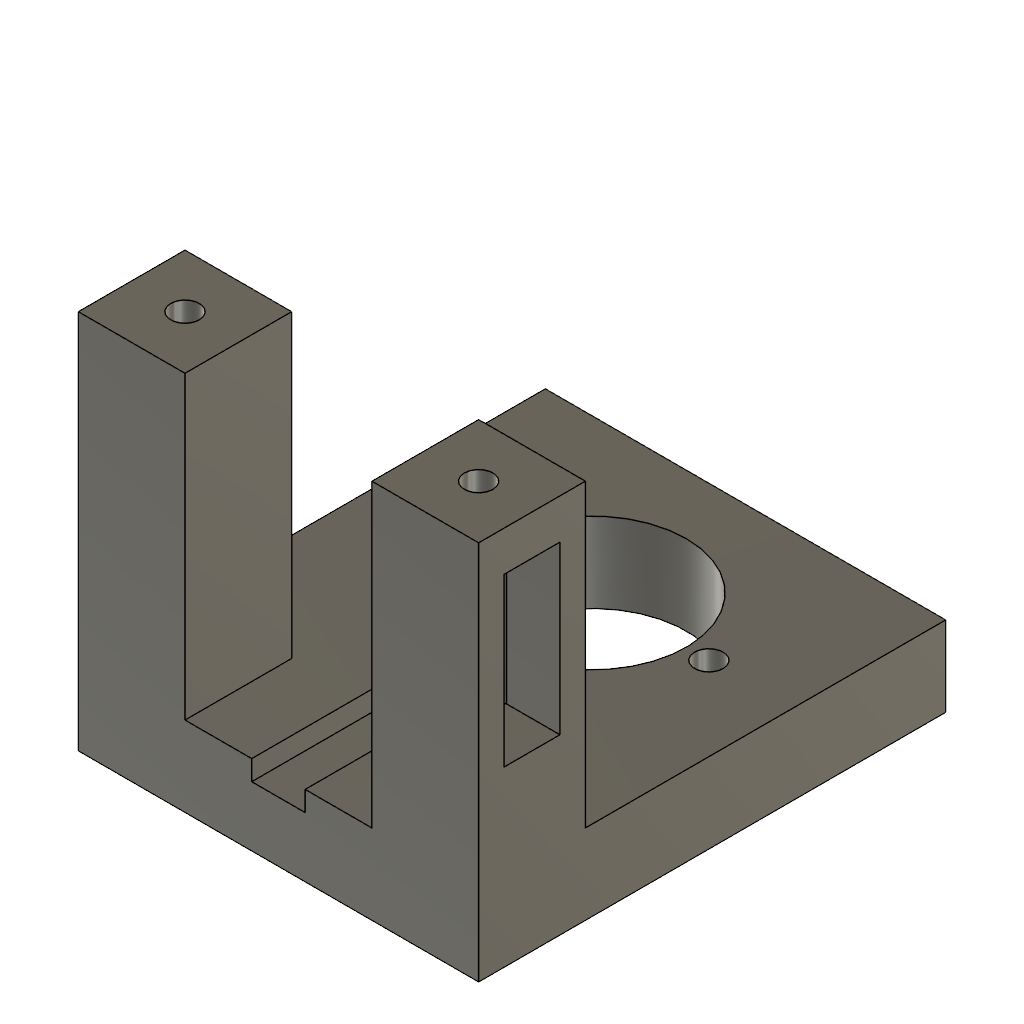
05 - PRIMARY SUPPORT MECHANISM ( LEFT SIDE ) (Autodesk Fusion 360 design; units mm, degrees)
Autodesk Fusion 360 part; units mm, degrees
sketch "01 - PRIMARY SUPPORT MECHANISM ( LEFT SIDE ) SKETCH" plane through (0, 0, 0) normal (0, 0, 1) x (1, 0, 0)
  line L0 (0, -35) -> (0, -5.422) construction
  line L1 (13.875, 9.9067) -> (17.5, 7.8138)
  circle A0 centre (17.5, 11.9996) radius 2.14
  line L2 (-13.875, 14.0925) -> (-17.5, 16.1854)
  circle A1 centre (-17.5, 11.9996) radius 2.14
  line L3 (-21.125, 14.0925) -> (-21.125, 9.9067)
  line L4 (4, -5.422) -> (4, -35)
  line L5 (30, 35) -> (30, -35)
  line L6 (-7.6, -5.422) -> (-7.6, 0.1231)
  line L7 (-4, -5.422) -> (-4, -35)
  line L8 (17.5, 7.8138) -> (21.125, 9.9067)
  line L9 (-21.125, 9.9067) -> (-17.5, 7.8138)
  line L10 (7.6, -5.422) -> (7.6, 0.1231)
  line L11 (21.125, 14.0925) -> (17.5, 16.1854)
  line L12 (-30, 35) -> (30, 35)
  line L13 (21.125, 9.9067) -> (21.125, 14.0925)
  line L14 (13.875, 14.0925) -> (13.875, 9.9067)
  line L15 (-17.5, 7.8138) -> (-13.875, 9.9067)
  line L16 (-30, -19) -> (30, -19) construction
  line L17 (30, -35) -> (-30, -35)
  line L18 (17.5, 16.1854) -> (13.875, 14.0925)
  line L19 (-17.5, 11.9996) -> (-17.5, 14.1396) construction
  line L20 (17.5, 11.9996) -> (17.5, 14.1396) construction
  line L21 (-17.5, 11.9996) -> (17.5, 11.9996) construction
  arc A2 (7.6, 0.1231) -> (-7.6, 0.1231) centre (0, 11.9996) ccw
  line L22 (-17.5, 16.1854) -> (-21.125, 14.0925)
  line L23 (-30, -35) -> (-30, 35)
  line L24 (-7.6, -5.422) -> (7.6, -5.422)
  line L25 (-13.875, 9.9067) -> (-13.875, 14.0925)
  point P0 (17.5, 11.9996)
  point P1 (-17.5, 11.9996)
  dimension "d1" = 60
  dimension "d2" = 70
  dimension "d5" = 16
  dimension "d6" = 29.578
  dimension "d7" = 15.2
  dimension "d8" = 5.5451
  dimension "d9" = 14.1
  dimension "d10" = 17.4216
  dimension "d11" = 8
  dimension "d12" = 4
  dimension "d13" = 35
  dimension "d14" = 4.28
  dimension "d15" = 3.625
  dimension "d16" = 4.28
  dimension "d17" = 3.625
  dimension "d19" = 35
  dimension "d20" = 30
  constraint horizontal L12
  constraint vertical L5
  constraint horizontal L17
  constraint vertical L23
  constraint coincident L16.start L23
  constraint coincident L16.end L5
  constraint perpendicular L5 L16
  constraint midpoint L0.start L17
  constraint perpendicular L0 L16
  constraint equal L6 L10
  constraint parallel L6 L10
  constraint perpendicular L10 L24
  constraint coincident L0.end L24
  constraint midpoint L0.end L24
  constraint horizontal L24
  constraint coincident L4.start L24
  constraint coincident L4.end L17
  constraint perpendicular L4 L17
  constraint coincident L7.start L24
  constraint coincident L7.end L17
  constraint perpendicular L7 L17
  constraint horizontal L21
  constraint midpoint A2.centre L21
  constraint coincident P0 A0.centre
  constraint coincident L20.end A0
  constraint perpendicular L20 L21
  constraint coincident L11.end L20
  constraint coincident P1 A1.centre
  constraint coincident L19.end A1
  constraint perpendicular L19 L21
  constraint coincident L2.end L19
  measures "d1" distance of L5.start L12.start
  measures "d2" distance of L12.start L17.end
  measures "d5" distance of L16 L17
  measures "d6" distance of L0.start L0.end
  measures "d7" distance of L10.start L6.start
  measures "d8" distance of L10.end L10.start
  measures "d9" radius of A2
  measures "d10" distance of A2.centre L24
  measures "d11" distance of L4 L7
  measures "d12" distance of L0 L7
  measures "d13" horizontal distance of P1 P0
  measures "d14" diameter of A0
  measures "d15" distance of P0 L13
  measures "d16" diameter of A1
  measures "d17" distance of P1 L15
  measures "d19" distance of origin L12
  measures "d20" distance of origin L23
  measures "d38" distance of L4.start
extrude "Extrude1" add sketch "01 - PRIMARY SUPPORT MECHANISM ( LEFT SIDE ) SKETCH" along normal blind 12 contours L1 L8 L11 L13 L18 A2 | L1 L2 L3 L4 L5 L6 L7 L8 L9 L10 L11 L12 L13 L15 L17 L18 A2 L22 L23 L24 | L2 L3 L9 L15 A2 L22 | A0 | A1
extrude "Extrude2" add sketch "01 - PRIMARY SUPPORT MECHANISM ( LEFT SIDE ) SKETCH" along normal blind 9 contours L4 L7 L17 L24
sketch "02 - PRIMARY SUPPORT MECHANISM ( LEFT SIDE ) SKETCH" plane through (0, 0, 12) normal (0, 0, 1) x (-1, 0, 0)
  line L0 (-4, 5.422) -> (-4, 35)
  line L1 (-4, 35) -> (-30, 35)
  line L2 (-30, 35) -> (-30, -35)
  line L3 (-30, -35) -> (30, -35)
  line L4 (30, -35) -> (30, 35)
  line L5 (30, 35) -> (4, 35)
  line L6 (4, 35) -> (4, 5.422)
  line L7 (4, 5.422) -> (7.6, 5.422)
  line L8 (7.6, 5.422) -> (7.6, -0.1231)
  arc A0 (-7.6, -0.1231) -> (7.6, -0.1231) centre (0, -11.9996) ccw
  line L9 (-7.6, -0.1231) -> (-7.6, 5.422)
  line L10 (-7.6, 5.422) -> (-4, 5.422)
  line L11 (30, 35) -> (4, 35)
  line L12 (-4, 35) -> (-30, 35)
  line L13 (30, 35) -> (14, 35)
  line L14 (-14, 35) -> (-14, 19)
  line L15 (14, 35) -> (14, 19)
  line L16 (-30, 19) -> (-30, 35)
  line L17 (-30, 35) -> (-14, 35)
  line L18 (30, 19) -> (30, 35)
  line L19 (14, 19) -> (30, 19)
  line L20 (-14, 19) -> (-30, 19)
  dimension "d25" = 16
  dimension "d26" = 16
  dimension "d27" = 16
  dimension "d28" = 16
  constraint horizontal L13
  constraint vertical L15
  constraint horizontal L19
  constraint vertical L18
  constraint coincident L4.end L5.start
  constraint horizontal L17
  constraint vertical L14
  constraint horizontal L20
  constraint vertical L16
  constraint coincident L1.end L2.start
  constraint coincident L5.end L6.start
  constraint coincident L0.end L1.start
  measures "d25" distance of L13.end L4.end
  measures "d26" distance of L18.start L4.end
  measures "d27" distance of L14.start L1.end
  measures "d28" distance of L1.end L16.start
extrude "Extrude3" add sketch "02 - PRIMARY SUPPORT MECHANISM ( LEFT SIDE ) SKETCH" along normal blind 45 contours L1 L2 L12 L14 L16 L17 L20 | L4 L5 L11 L13 L15 L18 L19
sketch "03 - PRIMARY SUPPORT MECHANISM ( LEFT SIDE ) SKETCH" plane through (0, 0, 57) normal (0, 0, 1) x (-1, 0, 0)
  line L0 (-14, 19) -> (-14, 35)
  line L1 (-14, 35) -> (-30, 35)
  line L2 (-30, 35) -> (-30, 19)
  line L3 (-30, 19) -> (-14, 19)
  line L4 (-14, 35) -> (-30, 35)
  line L5 (-18.375, 29.0929) -> (-22, 31.1858)
  line L6 (-14, 19) -> (-14, 35)
  line L7 (-22, 22.8142) -> (-18.375, 24.9071)
  line L8 (-14, 27) -> (-30, 27) construction
  line L9 (-25.625, 29.0929) -> (-25.625, 24.9071)
  line L10 (-30, 19) -> (-14, 19)
  line L11 (-22, 23.375) -> (-22, 22.8142)
  line L12 (-25.625, 24.9071) -> (-22, 22.8142)
  line L13 (-22, 22.8142) -> (-30, 22.8142)
  line L14 (-18.375, 24.9071) -> (-18.375, 29.0929)
  line L15 (-22, 31.1858) -> (-22, 30.625)
  line L16 (-30, 31.1858) -> (-30, 22.8142)
  line L17 (-30, 35) -> (-30, 19)
  line L18 (-22, 31.1858) -> (-25.625, 29.0929)
  line L19 (-22, 31.1858) -> (-30, 31.1858)
  circle A0 centre (-22, 27) radius 2.14
  line L20 (-22, 19) -> (-22, 35) construction
  point P0 (-22, 27)
  dimension "d34" = 3.625
  dimension "d35" = 4.28
  dimension "d38" = 16
  dimension "d39" = 16
  constraint midpoint L8.start L6
  constraint midpoint L8.end L17
  constraint midpoint L20.start L10
  constraint midpoint L20.end L4
  constraint midpoint P0 L8
  constraint coincident L5.end L20
  constraint coincident L13.end L17
  constraint perpendicular L13 L17
  constraint coincident L16.start L17
  constraint perpendicular L17 L19
  constraint coincident L11.start L20
  constraint coincident L15.end L20
  constraint coincident P0 A0.centre
  constraint coincident L1.end L2.start
  constraint coincident L0.end L1.start
  constraint coincident L2.end L3.start
  measures "d34" distance of P0 L9
  measures "d35" diameter of A0
  measures "d38" distance of L2.end L0.start
  measures "d39" distance of L0.end L0.start
extrude "Extrude4" cut sketch "03 - PRIMARY SUPPORT MECHANISM ( LEFT SIDE ) SKETCH" against normal blind 25 from surface at -6 contours L2 L9 L12 L13 L16 L17 L18 L19 | L5 L7 L9 L12 L14 L18 | A0
extrude "Extrude5" cut sketch "03 - PRIMARY SUPPORT MECHANISM ( LEFT SIDE ) SKETCH" against normal blind 6 contours A0
sketch "04 - PRIMARY SUPPORT MECHANISM ( LEFT SIDE ) SKETCH" plane through (0, 0, 57) normal (0, 0, 1) x (-1, 0, 0)
  line L0 (14, 19) -> (30, 19)
  line L1 (30, 19) -> (30, 35)
  line L2 (30, 35) -> (14, 35)
  line L3 (14, 35) -> (14, 19)
  line L4 (22, 35) -> (22, 19) construction
  line L5 (30, 27) -> (14, 27) construction
  line L6 (22, 31.1858) -> (18.375, 29.0929)
  line L7 (18.375, 24.9071) -> (22, 22.8142)
  line L8 (30, 35) -> (14, 35)
  line L9 (22, 22.8142) -> (30, 22.8142)
  line L10 (30, 19) -> (30, 35)
  line L11 (25.625, 29.0929) -> (22, 31.1858)
  line L12 (30, 31.1858) -> (30, 22.8142)
  line L13 (22, 22.8142) -> (25.625, 24.9071)
  circle A0 centre (22, 27) radius 2.14
  line L14 (18.375, 29.0929) -> (18.375, 24.9071)
  line L15 (22, 31.1858) -> (30, 31.1858)
  line L16 (25.625, 24.9071) -> (25.625, 29.0929)
  line L17 (14, 19) -> (30, 19)
  line L18 (14, 35) -> (14, 19)
  point P0 (22, 27)
  dimension "d47" = 3.625
  dimension "d48" = 4.28
  dimension "d49" = 16
  dimension "d50" = 16
  constraint midpoint L5.start L10
  constraint midpoint L5.end L18
  constraint midpoint L4.start L8
  constraint midpoint L4.end L17
  constraint midpoint P0 L4
  constraint coincident L6.start L4
  constraint coincident P0 A0.centre
  constraint coincident L9.end L10
  constraint perpendicular L9 L10
  constraint coincident L12.start L10
  constraint perpendicular L10 L15
  constraint coincident L1.end L2.start
  constraint coincident L2.end L3.start
  constraint coincident L0.end L1.start
  measures "d47" distance of P0 L14
  measures "d48" diameter of A0
  measures "d49" distance of L0.end L0.start
  measures "d50" distance of L2.end L0.start
extrude "Extrude6" cut sketch "04 - PRIMARY SUPPORT MECHANISM ( LEFT SIDE ) SKETCH" against normal blind 25 from surface at -6 contours L1 L9 L10 L11 L12 L13 L15 L16 | L6 L7 L11 L13 L14 L16 | A0
extrude "Extrude7" cut sketch "04 - PRIMARY SUPPORT MECHANISM ( LEFT SIDE ) SKETCH" against normal blind 6 contours A0
extrude "Extrude8" cut sketch "01 - PRIMARY SUPPORT MECHANISM ( LEFT SIDE ) SKETCH" along normal blind 12 contours A0 | A1
extrude "Extrude9" cut sketch "01 - PRIMARY SUPPORT MECHANISM ( LEFT SIDE ) SKETCH" along normal blind 4 contours L1 L8 L11 L13 L18 A2 | L2 L3 L9 L15 A2 L22
named bodies: "01 - PRIMARY SUPPORT MECHANISM ( LEFT SIDE )"
